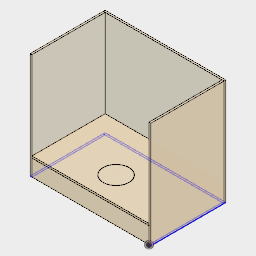
TurnTable (Autodesk Fusion 360 design; units mm, degrees)
Autodesk Fusion 360 part; units mm, degrees
note: some values were not read from the file. Chosen so that the rebuilt part matches the saved one: which bodies a step acts on.
sketch "スケッチ1" plane through (0, 0, 0) normal (0, 1, 0) x (1, 0, 0)
  line L0 (0, 0) -> (-787.4, 0)
  line L1 (-787.4, 0) -> (-787.4, 482.6)
  line L2 (-787.4, 482.6) -> (0, 482.6)
  line L3 (0, 482.6) -> (0, 0)
  line L4 (-800.1, 0) -> (12.7, 0)
  line L5 (12.7, 0) -> (12.7, -12.7)
  line L6 (12.7, -12.7) -> (-800.1, -12.7)
  line L7 (-800.1, -12.7) -> (-800.1, 0)
  line L8 (0, 482.6) -> (12.7, 482.6)
  line L9 (12.7, 482.6) -> (12.7, 0)
  line L10 (12.7, 0) -> (0, 0)
  line L11 (0, 0) -> (0, 482.6)
  line L12 (-800.1, 0) -> (-787.4, 0)
  line L13 (-787.4, 0) -> (-787.4, 482.6)
  line L14 (-787.4, 482.6) -> (-800.1, 482.6)
  line L15 (-800.1, 482.6) -> (-800.1, 0)
  line L16 (-800.1, 482.6) -> (12.7, 482.6)
  line L17 (12.7, 482.6) -> (12.7, 495.3)
  line L18 (12.7, 495.3) -> (-800.1, 495.3)
  line L19 (-800.1, 495.3) -> (-800.1, 482.6)
  dimension "d57" = 787.4
  dimension "d58" = 482.6
  dimension "d59" = 812.8
  dimension "d60" = 12.7
  dimension "d61" = 12.7
  dimension "d62" = 482.6
  dimension "d63" = 482.6
  dimension "d64" = 12.7
  dimension "d65" = 812.8
  measures "d57" distance of L0.start L0.end
  measures "d58" distance of L0.start L2.end
  measures "d59" distance of L4.start L4.end
  measures "d60" distance of L4.start L6.end
  measures "d61" distance of L2.end L8.end
  measures "d62" distance of L2.end L0.start
  measures "d63" distance of L4.start L14.end
  measures "d64" distance of L14.end L18.end
  measures "d65" distance of L14.end L8.end
combine "結合1" [no effect]
extrude "押し出し20" add sketch "スケッチ1" along normal blind 12.7 contours L0 L1 L2 L3 L4 L11 L13 L16 makes body 1
extrude "押し出し21" add sketch "スケッチ1" along normal blind 114.3 separate body contours L1 L4 L12 L13 L14 L15 L16 makes body 2
extrude "押し出し22" add sketch "スケッチ1" along normal blind 114.3 separate body contours L0 L4 L5 L6 L7 L10 L12 makes body 3
extrude "押し出し23" add sketch "スケッチ1" along normal blind 114.3 separate body contours L2 L8 L14 L16 L17 L18 L19 makes body 4
extrude "押し出し24" add sketch "スケッチ1" along normal blind 114.3 separate body contours L3 L4 L8 L9 L10 L11 L16 makes body 5
ref_plane "作業平面2" through (-393.7, 114.3, -488.95) normal (0, 1, 0) x (0, 0, 1)
sketch "スケッチ6" plane through (-393.7, 114.3, -488.95) normal (0, 1, 0) x (1, 0, 0)
  line L0 (-406.4, 6.35) -> (406.4, 6.35)
  line L1 (406.4, 6.35) -> (406.4, -501.65)
  line L2 (406.4, -501.65) -> (-406.4, -501.65)
  line L3 (-406.4, -501.65) -> (-406.4, 6.35)
  point P0 (-406.4, 6.35)
  dimension "d77" = 812.8
  dimension "d78" = 508
  measures "d77" distance of P0 L0.end
  measures "d78" distance of P0 L2.end
extrude "押し出し25" add sketch "スケッチ6" along normal blind 12.7 separate body makes body 6
sketch "スケッチ7" plane through (0, 0, 0) normal (0, 1, 0) x (1, 0, 0)
  line L0 (12.7, -12.7) -> (25.4, -12.7)
  line L1 (25.4, -12.7) -> (25.4, 495.3)
  line L2 (25.4, 495.3) -> (12.7, 495.3)
  line L3 (12.7, 495.3) -> (12.7, -12.7)
  line L4 (25.4, 495.3) -> (-812.8, 495.3)
  line L5 (-812.8, 495.3) -> (-812.8, 508)
  line L6 (-812.8, 508) -> (25.4, 508)
  line L7 (25.4, 508) -> (25.4, 495.3)
  line L8 (-812.8, 495.3) -> (-800.1, 495.3)
  line L9 (-800.1, 495.3) -> (-800.1, -12.7)
  line L10 (-800.1, -12.7) -> (-812.8, -12.7)
  line L11 (-812.8, -12.7) -> (-812.8, 495.3)
  point P0 (12.7, -12.7)
  dimension "d81" = 12.7
  dimension "d82" = 508
  dimension "d83" = 838.2
  dimension "d84" = 12.7
  dimension "d85" = 12.7
  dimension "d86" = 508
  measures "d81" distance of P0 L0.end
  measures "d82" distance of P0 L2.end
  measures "d83" distance of L1.end L4.end
  measures "d84" distance of L1.end L6.end
  measures "d85" distance of L4.end L8.end
  measures "d86" distance of L4.end L10.end
extrude "押し出し26" add sketch "スケッチ7" along normal blind 736.6 separate body contours L4 L8 L9 L10 L11 makes body 7
extrude "押し出し27" add sketch "スケッチ7" along normal blind 736.6 separate body contours L2 L4 L5 L6 L7 L8 makes body 8
extrude "押し出し28" add sketch "スケッチ7" along normal blind 736.6 separate body contours L0 L1 L2 L3 L4 makes body 9
sketch "スケッチ1 (2)" plane through (-812.8, 0, 0) normal (-1, 0, 0) x (0, 0, 1) in component "Sketches"
  line L0 (-495.3, 0) -> (12.7, 0)
  line L1 (12.7, 0) -> (12.7, 736.6)
  line L2 (12.7, 736.6) -> (-495.3, 736.6)
  line L3 (-495.3, 736.6) -> (-495.3, 0)
sketch "スケッチ2" plane through (0, 0, -508) normal (0, 0, -1) x (-1, 0, 0) in component "Sketches"
  line L0 (-25.4, 0) -> (812.8, 0)
  line L1 (812.8, 0) -> (812.8, 736.6)
  line L2 (812.8, 736.6) -> (-25.4, 736.6)
  line L3 (-25.4, 736.6) -> (-25.4, 0)
sketch "スケッチ3" plane through (25.4, 0, 0) normal (1, 0, 0) x (0, 0, -1) in component "Sketches"
  line L0 (-12.7, 0) -> (495.3, 0)
  line L1 (495.3, 0) -> (495.3, 736.6)
  line L2 (495.3, 736.6) -> (-12.7, 736.6)
  line L3 (-12.7, 736.6) -> (-12.7, 0)
sketch "スケッチ4" plane through (0, 127, 0) normal (0, 1, 0) x (-1, 0, 0) in component "Sketches"
  line L0 (800.1, 12.7) -> (-12.7, 12.7)
  line L1 (-12.7, 12.7) -> (-12.7, -495.3)
  line L2 (-12.7, -495.3) -> (800.1, -495.3)
  line L3 (800.1, -495.3) -> (800.1, 12.7)
sketch "スケッチ5" plane through (0, 0, 12.7) normal (0, 0, 1) x (1, 0, 0) in component "Sketches"
  line L0 (-800.1, 0) -> (12.7, 0)
  line L1 (12.7, 0) -> (12.7, 114.3)
  line L2 (12.7, 114.3) -> (-800.1, 114.3)
  line L3 (-800.1, 114.3) -> (-800.1, 0)
sketch "スケッチ6 (2)" plane through (-800.1, 0, 0) normal (-1, 0, 0) x (0, 0, 1) in component "Sketches"
  line L0 (-482.6, 0) -> (0, 0)
  line L1 (0, 0) -> (0, 114.3)
  line L2 (0, 114.3) -> (-482.6, 114.3)
  line L3 (-482.6, 114.3) -> (-482.6, 0)
sketch "スケッチ7 (2)" plane through (0, 0, -495.3) normal (0, 0, -1) x (-1, 0, 0) in component "Sketches"
  line L0 (-12.7, 0) -> (800.1, 0)
  line L1 (800.1, 0) -> (800.1, 114.3)
  line L2 (800.1, 114.3) -> (-12.7, 114.3)
  line L3 (-12.7, 114.3) -> (-12.7, 0)
sketch "スケッチ8" plane through (12.7, 0, 0) normal (1, 0, 0) x (0, 0, -1) in component "Sketches"
  line L0 (0, 0) -> (482.6, 0)
  line L1 (482.6, 0) -> (482.6, 114.3)
  line L2 (482.6, 114.3) -> (0, 114.3)
  line L3 (0, 114.3) -> (0, 0)
sketch "スケッチ9" plane through (0, 0, 0) normal (0, -1, 0) x (1, 0, 0) in component "Sketches"
  line L0 (0, -482.6) -> (0, 0)
  line L1 (0, 0) -> (-787.4, 0)
  line L2 (-787.4, 0) -> (-787.4, -482.6)
  line L3 (-787.4, -482.6) -> (0, -482.6)
sketch "スケッチ8 (2)" plane through (0, 127, 0) normal (0, 1, 0) x (-1, 0, 0)
  line L0 (800.1, 12.7) -> (-12.7, 12.7)
  line L1 (-12.7, 12.7) -> (-12.7, -495.3)
  line L2 (-12.7, -495.3) -> (800.1, -495.3)
  line L3 (800.1, -495.3) -> (800.1, 12.7)
  circle A0 centre (393.7, -165.1) radius 88.9
  circle A1 centre (393.7, -165.1) radius 90.4875
  dimension "d94" = 177.8
  dimension "d95" = 180.975
  measures "d94" diameter of A0
  measures "d95" diameter of A1
extrude "押し出し29" cut sketch "スケッチ8 (2)" against normal blind 25.4 contours A1 bodies 6 makes body 10 at (-694.4589, 114.3, -220.3955)
copy_body "ボディ -> コンポーネント1" [suppressed] in component "Component"
component "Sketches" placed x (1, 0, 0) y (0, 1, 0) z (0, 0, 1) at (0, 0, 0)
